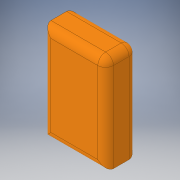
# Autodesk Inventor part: Motor Controller
Saved by Autodesk Inventor 2019 (Build 230136000, 136)
## iProperties
Created: 2019-02-21
Part Number: Motor Controller
Material: Generic
Document SubType Name: Modeling
Designer: varun
Density: 1 g/cm^3
Appearance: Orange
Author: varun
Autodesk Inventor part; units mm, degrees
ref_plane "YZ Plane" through (0, 0, 0) normal (1, 0, 0) x (0, 1, 0)
ref_plane "XZ Plane" through (0, 0, 0) normal (0, 1, 0) x (-1, 0, 0)
ref_plane "XY Plane" through (0, 0, 0) normal (0, 0, 1) x (1, 0, 0)
sketch "Sketch1" plane through (0, 0, 0) normal (0, 0, 1) x (1, 0, 0)
  line L0 (-6.35, -9.861) -> (6.35, -9.861)
  line L1 (6.35, -9.861) -> (6.35, 9.861)
  line L2 (6.35, 9.861) -> (-6.35, 9.861)
  line L3 (-6.35, 9.861) -> (-6.35, -9.861)
  line L4 (-6.35, -9.861) -> (6.35, 9.861) construction
  line L5 (6.35, -9.861) -> (-6.35, 9.861) construction
  point P0 (0, 0)
  dimension "d0" = 12.7
  constraints: 12 end point, 2 midpoint, 2 parallel, 1 horizontal, 1 perpendicular
  measures "d0" distance of L2.end L1.end
extrude "Extrusion1" add sketch "Sketch1" along normal blind 6.35
fillet "Fillet1" radius 1.5875 9 edges at (6.35, 0, 6.35) (6.35, 9.861, 3.175) (0, 9.861, 6.35) (0, 9.861, 0) (6.35, 0, 0) (0, -9.861, 6.35) (0, -9.861, 0) (-6.35, 0, 0) (-6.35, 0, 6.35)
body "Solid1"
